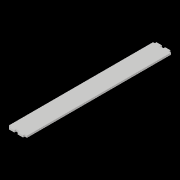
# Autodesk Inventor part: Top Shelf V3
Saved by Autodesk Inventor 2018 (Build 220112000, 112)
## iProperties
Created: 2017-09-13
Part Number: Top Shelf V3
Material: Generic
Document SubType Name: Modeling
Designer: gaine
Density: 1 g/cm^3
Appearance: Default
Author: gaine
Autodesk Inventor part; units mm, degrees
ref_plane "YZ Plane" through (0, 0, 0) normal (1, 0, 0) x (0, 1, 0)
ref_plane "XZ Plane" through (0, 0, 0) normal (0, 1, 0) x (-1, 0, 0)
ref_plane "XY Plane" through (0, 0, 0) normal (0, 0, 1) x (1, 0, 0)
sketch "Sketch1" plane through (0, 0, 0) normal (0, 1, 0) x (-1, 0, 0)
  line L0 (3.0163, -14.8736) -> (3.0163, -543.1936)
  line L1 (68.4721, -543.1936) -> (68.4721, -14.8736)
  line L2 (62.1221, -8.5236) -> (62.1221, -14.8736)
  line L3 (62.1221, -14.8736) -> (68.4721, -14.8736)
  line L4 (30.3721, -8.5236) -> (30.3721, -14.8736)
  line L5 (30.3721, -14.8736) -> (43.0721, -14.8736)
  line L6 (43.0721, -14.8736) -> (43.0721, -8.5236)
  line L7 (62.1221, -8.5236) -> (43.0721, -8.5236)
  line L8 (30.3721, -8.5236) -> (11.3221, -8.5236)
  line L9 (11.3221, -8.5236) -> (11.3221, -14.8736)
  line L10 (11.3221, -14.8736) -> (3.0163, -14.8736)
  line L11 (62.1221, -549.5436) -> (62.1221, -543.1936)
  line L12 (62.1221, -543.1936) -> (68.4721, -543.1936)
  line L13 (62.1221, -549.5436) -> (43.0721, -549.5436)
  line L14 (43.0721, -549.5436) -> (43.0721, -543.1936)
  line L15 (62.1221, -543.1936) -> (62.1221, -549.5436)
  line L16 (30.3721, -549.5436) -> (11.3221, -549.5436)
  line L17 (11.3221, -549.5436) -> (11.3221, -543.1936)
  line L18 (30.3721, -543.1936) -> (30.3721, -549.5436)
  line L19 (43.0721, -543.1936) -> (30.3721, -543.1936)
  line L20 (11.3221, -549.5436) -> (30.3721, -549.5436)
  line L21 (43.0721, -549.5436) -> (62.1221, -549.5436)
  line L22 (11.3221, -543.1936) -> (3.0163, -543.1936)
  point P0 (0, 0)
  dimension "d6" = 65.4558
  dimension "d11" = 19.05
  dimension "d12" = 19.05
  dimension "d13" = 12.7
  dimension "d14" = 6.35
  dimension "d15" = 8.3058
  dimension "d16" = 6.35
  dimension "d17" = 6.35
  dimension "d26" = 8.3058
  dimension "d27" = 19.05
  dimension "d28" = 12.7
  dimension "d29" = 19.05
  dimension "d30" = 6.35
  dimension "d31" = 6.35
  dimension "d32" = 6.35
  dimension "d33" = 6.35
  dimension "d34" = 6.35
  dimension "d37" = 541.02
  constraints: 46 end point, 8 parallel, 5 perpendicular, 4 horizontal
  measures "d6" distance between parallel lines of L0 L1
  measures "d11" distance between parallel lines of L6 L2
  measures "d12" distance between parallel lines of L9 L4
  measures "d13" distance between parallel lines of L4 L6
  measures "d14" distance between parallel lines of L2 L1
  measures "d15" distance between parallel lines of L0 L9
  measures "d16" distance between parallel lines of L3 L7
  measures "d17" distance between parallel lines of L5 L8
  measures "d26" distance between parallel lines of L0 L17
  measures "d27" distance between parallel lines of L18 L17
  measures "d28" distance between parallel lines of L14 L18
  measures "d29" distance between parallel lines of L14 L11
  measures "d30" distance between parallel lines of L11 L1
  measures "d31" distance between parallel lines of L13 L12
  measures "d32" distance between parallel lines of L13 L19
  measures "d33" distance between parallel lines of L20 L19
  measures "d34" distance between parallel lines of L16 L22
  measures "d37" distance between parallel lines of L8 L16
extrude "Extrusion1" add sketch "Sketch1" along normal blind 6.35
body "Solid1"
